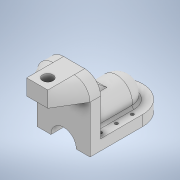
# Autodesk Inventor part: dhillg25_Graphics3
Saved by Autodesk Inventor 2021 (Build 250183000, 183)
## iProperties
Created: 2020-09-30
Part Number: dhillg25_Graphics3
Material: Generic
Document SubType Name: Modeling
Designer: gurle
Mass: 83.7836 g
Surface Area: 199.148 cm^2
Volume: 83.7836 cm^3
Density: 1 g/cm^3
Appearance: Default
Author: gurle
Autodesk Inventor part; units mm, degrees
ref_plane "XZ Plane" through (0, 0, 0) normal (0, 1, 0) x (-1, 0, 0)
sketch "Sketch1" plane through (0, 0, 0) normal (0, 1, 0) x (-1, 0, 0)
  line L0 (0, 0) -> (50, 0)
  line L1 (50, 0) -> (50, -40)
  line L2 (50, -40) -> (0, -40)
  line L3 (0, -40) -> (0, 0)
  arc A0 (0, -40) -> (50, -40) centre (25, -40) ccw
  line L4 (0, 0) -> (50, 0)
  line L5 (50, 0) -> (50, 10)
  line L6 (50, 10) -> (0, 10)
  line L7 (0, 10) -> (0, 0)
  dimension "d0" = 50
  dimension "d1" = 40
  dimension "d2" = 10
  dimension "d3" = 50
  constraints: 16 end point, 4 parallel, 2 horizontal, 2 perpendicular, 2 point on circle, 1 centre point, 1 midpoint
  measures "d0" distance of L1.end L2.end
  measures "d1" distance of L0.end L1.end
  measures "d2" distance of L5.end L4.end
  measures "d3" distance of L5.end L6.end
extrude "Extrusion1" add sketch "Sketch1" along normal blind 10
sketch "Sketch2" plane through (-50, 0, 10) normal (0, 0, 1) x (1, 0, 0)
  line L0 (0, 0) -> (0, 10) projected
  line L1 (0, 10) -> (50, 10)
  line L2 (50, 10) -> (50, 45)
  line L3 (35, 60) -> (15, 60)
  line L4 (0, 45) -> (0, 10)
  arc A0 (15, 60) -> (0, 45) centre (15, 45) ccw
  arc A1 (50, 45) -> (35, 60) centre (35, 45) ccw
  point P0 (50, 0)
  point P1 (50, 60)
  point P2 (0, 60)
  dimension "d6" = 50
  dimension "d7" = 50
  dimension "d8" = 15
  constraints: 8 end point, 4 point on circle, 4 point on line, 4 tangent, 2 centre point, 2 parallel, 1 equal radius, 1 horizontal, 1 perpendicular
  measures "d6" distance of L1.end point (50, 60)
  measures "d7" distance of point (50, 60) point (0, 60)
  measures "d8" radius of A0
extrude "Extrusion2" add sketch "Sketch2" against normal blind 10
sketch "Sketch3" plane through (-50, 0, 0) normal (0, 0, -1) x (-1, 0, 0)
  line L0 (-15, 60) -> (-35, 60) construction
  line L1 (-25, 60) -> (-25, 0) construction
  line L2 (0, 0) -> (-50, 0) construction
  circle A0 centre (-25, 15) radius 15
  dimension "d11" = 30
  dimension "d12" = 15
  constraints: 2 end point, 2 midpoint, 1 centre point, 1 point on line
  measures "d11" diameter of A0
  measures "d12" distance from line of L2 A0.centre
extrude "Extrusion3" add sketch "Sketch3" along normal blind 55
fillet "Fillet1" radius 15 1 edges at (-25, 30, -55)
fillet "Fillet2" radius 2 4 edges at (-35, 10, -50) (-15, 10, -50) (-39.1421, 10, -20) (-10.8579, 10, -20)
sketch "Sketch4" plane through (-50, 0, 10) normal (0, 0, 1) x (1, 0, 0)
  line L0 (0, 0) -> (50, 0) projected
  arc A0 (37, 0) -> (13, 0) centre (25, 0) ccw
  dimension "d17" = 24
  constraints: 2 point on circle, 2 point on line, 1 centre point, 1 midpoint
  measures "d17" diameter of A0
sketch "Sketch5" plane through (0, 10, 0) normal (0, 1, 0) x (1, 0, 0)
  circle A0 centre (-5, 5) radius 1.5
  line L0 (0, 0) -> (0, 40) projected
  line L1 (0, 0) -> (-15, 0) projected
  line L2 (-5, 5) -> (-5, 20) construction
  circle A1 centre (-5, 20) radius 1.5
  circle A2 centre (-5, 35) radius 1.5
  line L3 (-35, 0) -> (-15, 0) construction
  line L4 (-25, 0) -> (-25, 51.2461) construction
  circle A3 centre (-45, 5) radius 1.5
  circle A4 centre (-45, 20) radius 1.5
  circle A5 centre (-45, 35) radius 1.5
  dimension "d18" = 3
  dimension "d19" = 5
  dimension "d20" = 5
  dimension "d21" = 15
  dimension "d24" = 15
  constraints: 6 centre point, 4 end point, 3 symmetric about line, 3 vertical, 1 midpoint, 7 other
  measures "d18" diameter of A0
  measures "d19" distance from line of L0 L2.start
  measures "d20" distance from line of L1 L2.start
  measures "d21" distance of L2.start L2.end
  measures "d24" distance of L2.start A1.centre
extrude "Extrusion4" cut sketch "Sketch5" against normal blind 62
ref_plane "Work Plane1" through (-25, 0, 0) normal (1, 0, 0) x (0, 1, 0)
sketch "Sketch7" plane through (-25, 0, 0) normal (1, 0, 0) x (0, 1, 0)
  line L0 (30, 0) -> (30, -40) construction
  line L1 (30, 0) -> (30, -25) construction
  line L2 (30, -25) -> (26, -25) construction
  line L3 (26, -25) -> (26, -30) construction
  line L4 (30, 0) -> (12.3529, 0) construction
  line L5 (30, 0) -> (50, 0) construction
  line L6 (45, 0) -> (60, 0) construction
  line L7 (50, 0) -> (26, -30)
  line L8 (50, 0) -> (26, 0)
  line L9 (26, 0) -> (26, -30)
  point P0 (0, 0)
  dimension "d43" = 25
  dimension "d44" = 4
  dimension "d45" = 5
  dimension "d46" = 20
  constraints: 14 end point, 4 point on line, 2 perpendicular, 1 horizontal
  measures "d43" distance of L1.start L1.end
  measures "d44" distance of L1.end L2.end
  measures "d45" distance of L2.end L3.end
  measures "d46" distance of L1.start L5.end
extrude "Extrusion6" add sketch "Sketch7" along normal mid plane 10
sketch "Sketch8" plane through (-50, 0, 10) normal (0, 0, 1) x (1, 0, 0)
  line L0 (50, 45) -> (50, 10) projected
  line L1 (15, 60) -> (35, 60)
  line L2 (50, 45) -> (50, 45)
  line L3 (50, 45) -> (0, 45)
  line L4 (0, 45) -> (0, 45)
  arc A0 (50, 45) -> (35, 60) centre (35, 45) ccw
  arc A1 (15, 60) -> (0, 45) centre (15, 45) ccw
  point P0 (50, 0)
  point P1 (50, 60)
  dimension "d49" = 15
  dimension "d50" = 15
  constraints: 8 end point, 4 point on circle, 4 tangent, 2 centre point, 2 parallel, 2 point on line, 1 equal radius, 1 horizontal, 1 perpendicular
  measures "d49" distance of point (50, 60) L0.start
  measures "d50" radius of A0
ref_plane "Work Plane2" through (-50, 0, 35) normal (0, 0, 1) x (1, 0, 0)
sketch "Sketch9" plane through (-50, 0, 35) normal (0, 0, 1) x (1, 0, 0)
  line L0 (15, 60) -> (35, 60) projected
  line L1 (15, 60) -> (35, 60)
  line L2 (35, 60) -> (35, 45)
  line L3 (35, 45) -> (15, 45)
  line L4 (15, 45) -> (15, 60)
  point P0 (50, 0)
  dimension "d52" = 20
  dimension "d53" = 15
  constraints: 8 end point, 2 parallel, 1 horizontal, 1 perpendicular
  measures "d52" distance of L2.end L3.end
  measures "d53" distance of L1.end L2.end
loft "Loft1" add profiles "Sketch9", "Sketch8"
sketch "Sketch10" plane through (-35, 60, 0) normal (0, 1, 0) x (1, 0, 0)
  circle A0 centre (10, -25) radius 5
  line L0 (0, -35) -> (0, -10) projected
  line L1 (0, -35) -> (20, -35) projected
  point P0 (35, 0)
  dimension "d58" = 10
  dimension "d59" = 10
  dimension "d60" = 10
  constraints: 1 centre point
  measures "d58" diameter of A0
  measures "d59" distance from line of L0 A0.centre
  measures "d60" distance from line of L1 A0.centre
extrude "Extrusion7" cut sketch "Sketch10" against normal blind 62
extrude "Extrusion8" cut sketch "Sketch4" against normal blind 62
fillet "Fillet3" radius 12 1 edges at (-25, 12, -52)
body "Solid1"
